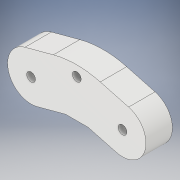
# Autodesk Inventor part: Body2
Saved by Autodesk Inventor 2017 SP1 (Build 210196100, 196)
## iProperties
Created: 2018-02-11
Part Number: Body2
Material: ABS Plastic
Document SubType Name: Modeling
Designer: Zach
Density: 1.06 g/cm^3
Appearance: CR White
Author: Zach
Autodesk Inventor part; units mm, degrees
ref_plane "YZ Plane" through (0, 0, 0) normal (1, 0, 0) x (0, 1, 0)
ref_plane "XZ Plane" through (0, 0, 0) normal (0, 1, 0) x (-1, 0, 0)
ref_plane "XY Plane" through (0, 0, 0) normal (0, 0, 1) x (1, 0, 0)
sketch "Sketch1" plane through (0, 0, 0) normal (0, 0, 1) x (1, 0, 0)
  line L0 (19.4476, -5.1392) -> (29.1069, -7.7274)
  line L1 (19.4476, -5.1392) -> (23.5887, 10.3156) construction
  line L2 (11.7298, -5.1392) -> (19.4476, -5.1392)
  line L3 (7.5887, 10.3156) -> (11.7298, -5.1392) construction
  line L4 (7.5887, 10.3156) -> (23.5887, 10.3156) construction
  arc A0 (23.5887, 10.3156) -> (7.5887, 10.3156) centre (15.5887, -19.5408) ccw
  line L5 (11.7298, -5.1392) -> (2.0706, -7.7274)
  line L6 (-2.0706, 7.7274) -> (7.5887, 10.3156)
  arc A1 (-2.0706, 7.7274) -> (2.0706, -7.7274) centre (0, 0) ccw
  circle A2 centre (0, 0) radius 8 construction
  circle A3 centre (31.1774, 0) radius 8 construction
  arc A4 (29.1069, -7.7274) -> (33.248, 7.7274) centre (31.1774, 0) ccw
  line L7 (23.5887, 10.3156) -> (33.248, 7.7274)
  circle A5 centre (0, 0) radius 1.5
  circle A6 centre (31.1774, 0) radius 1.5
  circle A7 centre (15.5887, 7.8608) radius 1.5
  point P0 (0, 0)
  point P1 (15.5887, 10.3156)
  dimension "d0" = 16
  dimension "d1" = 16
  dimension "d2" = 16
  dimension "d3" = 10
  dimension "d4" = 10
  dimension "d5" = 16
  dimension "d6" = 16
  dimension "d7" = 75
  dimension "d8" = 3
  dimension "d9" = 3
  dimension "d10" = 3
  dimension "d11" = 13
  constraints: 16 end point, 10 point on circle, 10 tangent, 8 centre point, 3 coincident, 2 horizontal alignment, 2 perpendicular, 1 horizontal, 1 midpoint, 1 point on line, 1 vertical alignment
  measures "d0" diameter of A3
  measures "d1" diameter of A2
  measures "d2" distance of L3.start L2.start
  measures "d3" distance from line of A2.centre L3
  measures "d4" distance from line of L1 A3.centre
  measures "d5" distance of L0.start L1.end
  measures "d6" distance of L3.start L1.end
  measures "d7" angle of L4 L3
  measures "d8" diameter of A5
  measures "d9" diameter of A6
  measures "d10" diameter of A7
  measures "d11" distance from line of L2 A7.centre
extrude "Extrusion1" add sketch "Sketch1" along normal blind 9
body "Solid1"
